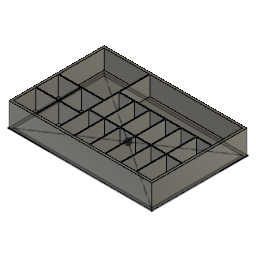
Semana4_Desafio4 v1 (Autodesk Fusion 360 design; units mm, degrees)
Autodesk Fusion 360 part; units mm, degrees
note: some values were not read from the file. Chosen so that the rebuilt part matches the saved one: where a step ends; a direction.
sketch "Sketch1" plane through (0, 0, 0) normal (0, 0, 1) x (1, 0, 0)
  line L0 (150, -100) -> (-150, -100)
  line L1 (-150, -100) -> (-150, 100)
  line L2 (-150, 100) -> (150, 100)
  line L3 (150, 100) -> (150, -100)
  line L4 (150, -100) -> (-150, 100) construction
  line L5 (-150, -100) -> (150, 100) construction
  line L6 (145, -95) -> (-145, -95)
  line L7 (-145, -95) -> (-145, 95)
  line L8 (-145, 95) -> (145, 95)
  line L9 (145, 95) -> (145, -95)
  line L10 (145, -95) -> (-145, 95) construction
  line L11 (-145, -95) -> (145, 95) construction
  dimension "d1" = 290
  dimension "d2" = 190
  dimension "d3" = 300
  dimension "d4" = 200
  constraint horizontal L0
  constraint perpendicular L0 L1
  constraint parallel L0 L2
  constraint parallel L1 L3
  constraint coincident L4 origin
  constraint coincident L5 origin
  constraint horizontal L6
  constraint perpendicular L6 L7
  constraint parallel L6 L8
  constraint parallel L7 L9
  constraint coincident L10 origin
  constraint coincident L11 origin
  measures "d1" distance of L7.end L8.end
  measures "d2" distance of L6.end L7.end
  measures "d3" distance of L1.end L2.end
  measures "d4" distance of L0.start L2.end
extrude "Extrude1" add sketch "Sketch1" along normal blind 50
extrude "Extrude2" add sketch "Sketch1" along normal blind 10 contours L6 L7 L8 L9
sketch "Sketch6" plane through (0, 0, 50) normal (0, 0, 1) x (-1, 0, 0)
  line L0 (145, -95) -> (-145, -95)
  line L1 (-145, -95) -> (-145, 95)
  line L2 (-145, 95) -> (145, 95)
  line L3 (145, 95) -> (145, -95)
  line L4 (-150, -100) -> (150, -100)
  line L5 (150, -100) -> (150, 100)
  line L6 (150, 100) -> (-150, 100)
  line L7 (-150, 100) -> (-150, -100)
  line L8 (50, -95) -> (50, 95)
  line L9 (50, 0) -> (145, 0)
  line L10 (50, -31) -> (-145, -31)
  line L11 (-145, 32) -> (50, 32)
  line L12 (17.5, -31) -> (17.5, 95)
  line L13 (-15, -31) -> (-15, 95)
  line L14 (-47.5, -31) -> (-47.5, 95)
  line L15 (-80, 95) -> (-80, -31)
  line L16 (-112.5, -31) -> (-112.5, 95)
  line L17 (97.5, 0) -> (97.5, 95)
  line L18 (145, 47.5) -> (50, 47.5)
  line L19 (145, 95) -> (145, -95)
  line L20 (-145, 95) -> (145, 95)
  line L21 (-145, -95) -> (-145, 95)
  dimension "d42" = 95
  dimension "d43" = 63
  dimension "d44" = 63
  dimension "d45" = 32.5
  dimension "d46" = 32.5
  dimension "d47" = 32.5
  dimension "d48" = 32.5
  dimension "d49" = 32.5
  constraint coincident L0 L8.start
  constraint coincident L2 L8.end
  constraint perpendicular L2 L8
  constraint midpoint L8 L9.start
  constraint midpoint L3 L9.end
  constraint coincident L8 L10.start
  constraint coincident L1 L10.end
  constraint perpendicular L1 L10
  constraint coincident L1 L11.start
  constraint coincident L8 L11.end
  constraint perpendicular L8 L11
  constraint coincident L10 L12.start
  constraint coincident L2 L12.end
  constraint perpendicular L2 L12
  constraint coincident L10 L13.start
  constraint coincident L2 L13.end
  constraint perpendicular L2 L13
  constraint coincident L10 L14.start
  constraint coincident L2 L14.end
  constraint perpendicular L2 L14
  constraint coincident L2 L15.start
  constraint coincident L10 L15.end
  constraint perpendicular L10 L15
  constraint coincident L10 L16.start
  constraint coincident L2 L16.end
  constraint perpendicular L2 L16
  constraint midpoint L9 L17.start
  constraint coincident L2 L17.end
  constraint perpendicular L2 L17
  constraint coincident L3 L18.start
  constraint coincident L8 L18.end
  constraint perpendicular L8 L18
  constraint midpoint L17 L18
  measures "d42" distance of L8 L19
  measures "d43" distance of L10 L11
  measures "d44" distance of L11 L20
  measures "d45" distance of L8 L12
  measures "d46" distance of L16 L21
  measures "d47" distance of L15 L16
  measures "d48" distance of L14 L15
  measures "d49" distance of L13 L14
rib "Web1" add thickness 2 on both sides direction (0, 0, -1) up to next path "Sketch6" along L8 L9 L18 L17 L12 L10 L11 L13 L14 L15 L16
